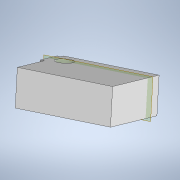
# Autodesk Inventor part: new slider part
Saved by Autodesk Inventor 2022 (Build 260153070, 153G)
## iProperties
Created: 2021-07-24
Part Number: new slider part
Material: Generic
Document SubType Name: Sheet Metal
Designer: DELL
Density: 1 g/cm^3
Sheet Metal Rule: Default
Appearance: Default
Author: DELL
Autodesk Inventor part; units mm, degrees
ref_plane "YZ Plane" through (0, 0, 0) normal (1, 0, 0) x (0, 1, 0)
ref_plane "XZ Plane" through (0, 0, 0) normal (0, 1, 0) x (-1, 0, 0)
ref_plane "XY Plane" through (0, 0, 0) normal (0, 0, 1) x (1, 0, 0)
sketch "Sketch1" plane through (0, 0, 0) normal (0, 0, 1) x (1, 0, 0)
  line L0 (-11.7555, 11.7555) -> (11.7555, 11.7555)
  line L1 (11.7555, 11.7555) -> (11.7555, -8.812)
  line L2 (8.812, -11.7555) -> (-8.812, -11.7555)
  line L3 (-11.7555, -8.812) -> (-11.7555, 11.7555)
  line L4 (-11.7555, 11.7555) -> (11.7555, -11.7555) construction
  line L5 (11.7555, 11.7555) -> (-11.7555, -11.7555) construction
  line L6 (11.7555, -11.7555) -> (8.812, -11.7555)
  line L7 (8.812, -11.7555) -> (8.812, -8.812)
  line L8 (8.812, -8.812) -> (11.7555, -8.812)
  line L9 (11.7555, -8.812) -> (11.7555, -11.7555)
  line L10 (-8.812, -11.7555) -> (-8.812, -8.812)
  line L11 (-8.812, -8.812) -> (-11.7555, -8.812)
  circle A0 centre (0, 0) radius 6.35
  point P0 (0, 0)
  dimension "d4" = 12.7
  constraints: 24 end point, 4 parallel, 2 horizontal, 2 midpoint, 2 perpendicular, 2 point on line, 1 centre point, 1 coincident
  measures "d4" diameter of A0
extrude "Extrusion1" add sketch "Sketch1" along normal blind 25.4 contours L0 L1 L8 L7 L2 L10 L11 L3
mirror "Mirror1" about plane through (0, 0, 0) normal (1, 0, 0)
sketch "Sketch3" plane through (-11.7555, -8.812, 0) normal (-1, 0, 0) x (0, 0, 1)
  circle A0 centre (12.3172, 9.3487) radius 5.08
  point P0 (0, 8.812)
  dimension "d13" = 10.16
  constraints: 1 centre point
  measures "d13" diameter of A0
extrude "Extrusion3" add sketch "Sketch3" along normal blind 10.16
sketch "Sketch4" plane through (-11.7555, 11.7555, 0) normal (0, 1, 0) x (1, 0, 0)
  line L0 (23.5109, 0) -> (23.5109, -25.4) projected
  line L1 (0, 0) -> (2.9435, 0) projected
  line L2 (23.5109, -25.4) -> (0, -25.4)
  line L3 (0, -25.4) -> (0, 0)
  line L4 (0, 0) -> (23.5109, 0)
  line L5 (23.5109, 0) -> (23.5109, -25.4)
  point P0 (11.7555, 0)
  point P1 (2.9435, 0)
  constraints: 8 end point, 2 parallel, 1 horizontal, 1 perpendicular
extrude "Extrusion4" add sketch "Sketch4" along normal blind 50.8
sketch "Sketch5" plane through (11.7555, -8.812, 25.4) normal (1, 0, 0) x (0, 0, -1)
  line L0 (25.4, 0) -> (0, 0) projected
  line L1 (25.4, 0) -> (25.4, 71.3674) projected
  line L2 (0, 0) -> (25.4, 0)
  line L3 (25.4, 0) -> (25.4, 71.3674)
  line L4 (25.4, 71.3674) -> (0, 71.3674)
  line L5 (0, 71.3674) -> (0, 0)
  point P0 (25.4, 8.812)
  constraints: 8 end point, 2 parallel, 1 horizontal, 1 perpendicular
extrude "Extrusion5" add sketch "Sketch5" along normal blind 25.4
ref_plane "Work Plane1" through (0, 0, 0) normal (1, 0, 0) x (0, 1, 0)
equation "\"BendRadius\" = Thickness"
equation "\"BendReliefWidth\" = Thickness"
equation "\"BendReliefDepth\" = 0.5 * Thickness"
equation "\"CornerReliefSize\" = 4 * Thickness"
equation "\"MinimumRemnant\" = 2 * Thickness"
equation "\"TransitionRadius\" = BendRadius"
equation "\"JacobiRadiusSize\" = BendRadius"
equation "\"GapSize\" = Thickness"
equation "\"Thickness\" = 3.048"
body "Solid1"
